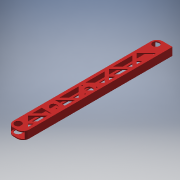
# Autodesk Inventor part: arm
Saved by Autodesk Inventor 2017 SP1 (Build 210196100, 196)
## iProperties
Created: 2018-01-23
Part Number: arm
Material: Aluminum 6061
Document SubType Name: Modeling
Designer: Ben
Density: 2.7 g/cm^3
Appearance: Light Red
Mass: 427.544 g
Surface Area: 1101.66 cm^2
Volume: 158.35 cm^3
Author: Ben
Autodesk Inventor part; units mm, degrees
ref_plane "YZ Plane" through (0, 0, 0) normal (1, 0, 0) x (0, 1, 0)
ref_plane "XZ Plane" through (0, 0, 0) normal (0, 1, 0) x (-1, 0, 0)
ref_plane "XY Plane" through (0, 0, 0) normal (0, 0, 1) x (1, 0, 0)
sketch "Sketch1" plane through (0, 0, 0) normal (0, 0, 1) x (1, 0, 0)
  line L0 (-25.4, -12.7) -> (25.4, -12.7)
  line L1 (25.4, -12.7) -> (25.4, 12.7)
  line L2 (25.4, 12.7) -> (-25.4, 12.7)
  line L3 (-25.4, 12.7) -> (-25.4, -12.7)
  line L4 (-25.4, -12.7) -> (25.4, 12.7) construction
  line L5 (25.4, -12.7) -> (-25.4, 12.7) construction
  line L6 (-22.225, -9.525) -> (22.225, -9.525)
  line L7 (22.225, -9.525) -> (22.225, 9.525)
  line L8 (22.225, 9.525) -> (-22.225, 9.525)
  line L9 (-22.225, 9.525) -> (-22.225, -9.525)
  line L10 (-22.225, -9.525) -> (22.225, 9.525) construction
  line L11 (22.225, -9.525) -> (-22.225, 9.525) construction
  line L12 (0, 9.525) -> (0, 12.7) construction
  line L13 (22.225, 0) -> (25.4, 0) construction
  point P0 (0, 0)
  dimension "d0" = 25.4
  dimension "d1" = 50.8
  dimension "d2" = 3.175
  constraints: 28 end point, 8 midpoint, 4 parallel, 3 perpendicular, 2 horizontal
  measures "d0" distance of L0.end L1.end
  measures "d1" distance of L1.end L2.end
  measures "d2" distance of L12.start L12.end
extrude "Extrusion1" add sketch "Sketch1" along normal blind 488.95
sketch "Sketch2" plane through (-25.4, 12.7, 0) normal (0, 1, 0) x (1, 0, 0)
  circle A0 centre (15.875, -469.9) radius 11.1379
  circle A1 centre (34.925, -257.3411) radius 11.1379
  circle A2 centre (25.4, -363.6206) radius 11.1379
  circle A3 centre (15.875, -19.05) radius 11.1125
  line L0 (0, 0) -> (0, -488.95) construction
  line L1 (3.175, 0) -> (3.175, -488.95) construction
  line L2 (50.8, 0) -> (50.8, -488.95) construction
  line L3 (15.875, -19.05) -> (24.1367, -26.4818) construction
  line L4 (15.875, -469.9) -> (34.925, -257.3411) construction
  line L5 (50.8, -488.95) -> (0, -488.95) projected
  line L6 (47.625, 0) -> (47.625, -488.95) construction
  circle A4 centre (41.275, -238.2911) radius 1.905
  circle A5 centre (41.275, -276.3911) radius 1.905
  circle A6 centre (12.7, -257.3411) radius 1.905
  line L7 (41.275, -238.2911) -> (41.275, -276.3911) construction
  line L8 (12.7, -257.3411) -> (47.625, -257.3411) construction
  circle A7 centre (34.925, -257.3411) radius 14.2875 construction
  point P0 (41.275, -257.3411)
  dimension "d10" = 22.225
  dimension "d5" = 22.2758
  dimension "d16" = 19.05
  dimension "d17" = 15.875
  dimension "d20" = 19.05
  dimension "d21" = 15.875
  dimension "d23" = 15.875
  dimension "d24" = 38.1
  dimension "d27" = 28.575
  dimension "d28" = 3.81
  dimension "d29" = 22.225
  dimension "d30" = 9.525
  dimension "d31" = 106.7054
  constraints: 8 end point, 7 centre point, 4 equal radius, 3 point on line, 2 coincident, 2 midpoint, 1 parallel, 1 perpendicular, 3 other
  measures "d5" diameter of A0
  measures "d16" vertical distance of L3.start L0.start
  measures "d17" distance from line of L0 L4.start
  measures "d20" distance from line of L5 L4.start
  measures "d21" distance from line of L0 L3.start
  measures "d23" distance from line of L2 L4.end
  measures "d24" distance of L7.start L7.end
  measures "d27" diameter of A7
  measures "d28" diameter of A6
  measures "d29" distance of L4.end L8.start
  measures "d30" distance between parallel lines of L2 L7
  measures "d31" distance of L4.start A2.centre
extrude "Extrusion2" cut sketch "Sketch2" against normal through all
fillet "Fillet1" radius 19.05 3 edges at (-25.4, 0, 0) (-25.4, 0, 488.95) (25.4, 0, 488.95)
sketch "Sketch3" plane through (-6.35, 12.7, 0) normal (0, 1, 0) x (1, 0, 0)
  arc A0 (12.7, -488.95) -> (31.75, -469.9) centre (12.7, -469.9) ccw construction
  line L0 (31.75, 0) -> (31.75, -469.9) construction
  line L1 (31.75, 0) -> (0, 0) construction
  arc A1 (0, 0) -> (-19.05, -19.05) centre (0, -19.05) ccw construction
  line L2 (-19.05, -19.05) -> (-19.05, -469.9) construction
  arc A2 (-19.05, -469.9) -> (0, -488.95) centre (0, -469.9) ccw construction
  line L3 (12.7, -488.95) -> (0, -488.95) construction
  circle A3 centre (6.35, -363.6206) radius 11.1379 construction
  circle A4 centre (-3.175, -469.9) radius 11.1379 construction
  circle A5 centre (22.225, -276.3911) radius 1.905 construction
  circle A6 centre (22.225, -238.2911) radius 1.905 construction
  circle A7 centre (-6.35, -257.3411) radius 1.905 construction
  circle A8 centre (15.875, -257.3411) radius 11.1379 construction
  circle A9 centre (-3.175, -19.05) radius 11.1125 construction
  line L4 (-9.525, -243.6112) -> (22.225, -211.8612)
  line L5 (22.225, -211.8612) -> (-9.525, -180.1112)
  line L6 (-9.525, -180.1112) -> (-9.525, -243.6112)
  line L7 (-9.525, -166.6408) -> (22.225, -198.3908)
  line L8 (22.225, -198.3908) -> (22.225, -134.8908)
  line L9 (22.225, -134.8908) -> (-9.525, -166.6408)
  line L10 (-9.525, -153.1704) -> (22.225, -121.4204)
  line L11 (22.225, -121.4204) -> (-9.525, -89.6704)
  line L12 (-9.525, -89.6704) -> (-9.525, -153.1704)
  line L13 (-9.525, -211.8612) -> (-19.05, -211.8612) construction
  line L14 (22.225, -211.8612) -> (31.75, -211.8612) construction
  line L15 (6.35, -195.9862) -> (13.0852, -189.251) construction
  line L16 (6.35, -150.7658) -> (-0.3852, -144.0306) construction
  line L17 (22.225, -107.95) -> (-9.525, -76.2)
  line L18 (-9.525, -76.2) -> (22.225, -44.45)
  line L19 (22.225, -44.45) -> (22.225, -107.95)
  line L20 (6.35, -105.5454) -> (13.0852, -98.8102) construction
  line L21 (-9.525, -431.5022) -> (22.225, -463.2522)
  line L22 (22.225, -463.2522) -> (22.225, -399.7522)
  line L23 (22.225, -399.7522) -> (-9.525, -431.5022)
  line L24 (-9.525, -418.0318) -> (22.225, -386.2818)
  line L25 (22.225, -386.2818) -> (-9.525, -386.2818)
  line L26 (-9.525, -386.2818) -> (-9.525, -418.0318)
  line L27 (6.35, -402.1568) -> (13.0852, -408.892) construction
  line L28 (6.35, -386.2818) -> (6.35, -374.7585) construction
  circle A10 centre (6.35, -363.6206) radius 11.1379 construction
  line L29 (12.8489, -453.8761) -> (4.7007, -462.0243) construction
  circle A11 centre (-3.175, -469.9) radius 11.1379 construction
  line L30 (-9.525, -265.8362) -> (22.225, -297.5862)
  line L31 (22.225, -297.5862) -> (-9.525, -329.3362)
  line L32 (-9.525, -329.3362) -> (-9.525, -265.8362)
  line L33 (-9.525, -342.8065) -> (22.225, -342.8065)
  line L34 (22.225, -342.8065) -> (22.225, -311.0565)
  line L35 (22.225, -311.0565) -> (-9.525, -342.8065)
  line L36 (6.35, -313.4612) -> (13.0852, -320.1963) construction
  circle A12 centre (15.875, -257.3411) radius 11.1379 construction
  point P0 (6.35, 0)
  dimension "d32" = 9.525
  dimension "d33" = 44.45
  dimension "d36" = 22.225
  constraints: 66 end point, 19 point on line, 16 equal length, 13 perpendicular, 7 midpoint, 6 parallel, 4 vertical, 3 collinear, 2 horizontal, 2 vertical alignment, 6 other
  measures "d32" distance of L13.start L13.end
  measures "d33" distance from line of L1 L18.end
  measures "d36" distance of L4.start L30.start
extrude "Extrusion3" cut sketch "Sketch3" against normal through all
body "Solid1"
